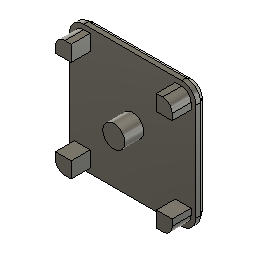
4040 end cap v7 (Autodesk Fusion 360 design; units mm, degrees)
Autodesk Fusion 360 part; units mm, degrees
sketch "Sketch1" plane through (0, 0, 0) normal (0, 0, 1) x (1, 0, 0)
  line L0 (15.5, -20) -> (-15.5, -20)
  line L1 (-20, -15.5) -> (-20, 15.5)
  line L2 (-15.5, 20) -> (15.5, 20)
  line L3 (20, 15.5) -> (20, -15.5)
  line L4 (15.5, 15.5) -> (-15.5, 15.5) construction
  line L5 (-15.5, 15.5) -> (-15.5, -15.5) construction
  line L6 (-15.5, -15.5) -> (15.5, -15.5) construction
  line L7 (15.5, -15.5) -> (15.5, 15.5) construction
  arc A0 (-20, -15.5) -> (-15.5, -20) centre (-15.5, -15.5) ccw
  arc A1 (15.5, -20) -> (20, -15.5) centre (15.5, -15.5) ccw
  arc A2 (20, 15.5) -> (15.5, 20) centre (15.5, 15.5) ccw
  arc A3 (-15.5, 20) -> (-20, 15.5) centre (-15.5, 15.5) ccw
  arc A4 (-18.5, -15.5) -> (-15.5, -18.5) centre (-15.5, -15.5) ccw
  circle A5 centre (0, 0) radius 3.5
  line L8 (-18.5, -15.5) -> (-18.5, -13.5)
  line L9 (-15.5, -18.5) -> (-13.5, -18.5)
  line L10 (-13.5, -18.5) -> (-13.5, -13.5)
  line L11 (-13.5, -13.5) -> (-18.5, -13.5)
  line L12 (18.5, -13.5) -> (13.5, -13.5)
  line L13 (13.5, -13.5) -> (13.5, -18.5)
  arc A6 (15.5, -18.5) -> (18.5, -15.5) centre (15.5, -15.5) ccw
  line L14 (15.5, -18.5) -> (13.5, -18.5)
  line L15 (18.5, -15.5) -> (18.5, -13.5)
  line L16 (13.5, 18.5) -> (13.5, 13.5)
  line L17 (13.5, 13.5) -> (18.5, 13.5)
  arc A7 (18.5, 15.5) -> (15.5, 18.5) centre (15.5, 15.5) ccw
  line L18 (18.5, 15.5) -> (18.5, 13.5)
  line L19 (15.5, 18.5) -> (13.5, 18.5)
  line L20 (-18.5, 13.5) -> (-13.5, 13.5)
  line L21 (-13.5, 13.5) -> (-13.5, 18.5)
  arc A8 (-15.5, 18.5) -> (-18.5, 15.5) centre (-15.5, 15.5) ccw
  line L22 (-15.5, 18.5) -> (-13.5, 18.5)
  line L23 (-18.5, 15.5) -> (-18.5, 13.5)
  dimension "d5" = 9
  dimension "d7" = 360
  dimension "d8" = 6
  dimension "d11" = 7
  dimension "d17" = 2
  dimension "d18" = 2
  dimension "d20" = 360
  constraint horizontal L0
  constraint perpendicular L0 L1
  constraint parallel L0 L2
  constraint parallel L1 L3
  constraint horizontal L4
  constraint perpendicular L4 L5
  constraint parallel L4 L6
  constraint parallel L5 L7
  constraint coincident L5.end L6.start
  constraint concentric A0 A4
  constraint coincident A5.centre origin
  constraint tangent A4 L8
  constraint perpendicular L9 L10
  measures "d5" diameter of A0
  measures "d8" diameter of A4
  measures "d11" diameter of A5
  measures "d17" distance of A4.start L8.end
  measures "d18" distance of A4.end L9.end
extrude "Extrude1" add sketch "Sketch1" along normal blind 3 contours L0 L1 L2 L3 A0 A1 A2 A3 | L12 L13 A6 L14 L15 | L16 L17 A7 L18 L19 | L20 L21 A8 L22 L23
extrude "Extrude2" add sketch "Sketch1" along normal blind 9 contours A4 L8 L9 L10 L11 | A5 | L12 L13 A6 L14 L15 | L16 L17 A7 L18 L19 | L20 L21 A8 L22 L23
chamfer "Chamfer1" distance 1 distance2 1.5 8 edges at (0, 20, 0) (18.682, 18.682, 0) (20, 0, 0) (18.682, -18.682, 0) (0, -20, 0) (-18.682, -18.682, 0) (-20, 0, 0) (-18.682, 18.682, 0) measured on face at (-6.6667, 5.1667, 0) measured on face at (15.7141, 19.9949, 2) measured on face at (-6.6667, 5.1667, 0) measured on face at (19.1656, -18.1103, 2) measured on face at (-6.6667, 5.1667, 0) measured on face at (-18.6054, -18.7568, 2) measured on face at (-6.6667, 5.1667, 0) measured on face at (-18.2817, 19.0372, 2)
